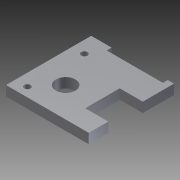
# Autodesk Inventor part: carro x lado motor pieza 2parte 2
Saved by Autodesk Inventor 2012 (Build 160160000, 160)
## iProperties
Created: 2014-12-17
Part Number: carro x lado motor pieza 2parte 2
Material: Default
Document SubType Name: Modeling
Designer: PRINCIPAL
Density: 1 g/cm^3
Author: PRINCIPAL
Autodesk Inventor part; units mm, degrees
ref_plane "YZ Plane" through (0, 0, 0) normal (1, 0, 0) x (0, 1, 0)
ref_plane "XZ Plane" through (0, 0, 0) normal (0, 1, 0) x (-1, 0, 0)
ref_plane "XY Plane" through (0, 0, 0) normal (0, 0, 1) x (1, 0, 0)
sketch "Boceto1" plane through (0, 0, 0) normal (0, 0, 1) x (1, 0, 0)
  arc A0 (-116.1173, -7.6512) -> (-117.6673, -9.2012) centre (-116.1173, -9.2012) ccw
  arc A1 (-117.6673, -9.2012) -> (-116.1173, -10.7512) centre (-116.1173, -9.2012) ccw
  arc A2 (-116.1173, -10.7512) -> (-114.5673, -9.2012) centre (-116.1173, -9.2012) ccw
  arc A3 (-114.5673, -9.2012) -> (-116.1173, -7.6512) centre (-116.1173, -9.2012) ccw
  arc A4 (-116.1173, -36.6512) -> (-117.6673, -38.2012) centre (-116.1173, -38.2012) ccw
  arc A5 (-117.6673, -38.2012) -> (-116.1173, -39.7512) centre (-116.1173, -38.2012) ccw
  arc A6 (-116.1173, -39.7512) -> (-114.5673, -38.2012) centre (-116.1173, -38.2012) ccw
  arc A7 (-114.5673, -38.2012) -> (-116.1173, -36.6512) centre (-116.1173, -38.2012) ccw
  arc A8 (-107.1173, -22.7512) -> (-112.0673, -27.7012) centre (-107.1173, -27.7012) ccw
  arc A9 (-112.0673, -27.7012) -> (-107.1173, -32.6512) centre (-107.1173, -27.7012) ccw
  arc A10 (-107.1173, -32.6512) -> (-102.1673, -27.7012) centre (-107.1173, -27.7012) ccw
  arc A11 (-102.1673, -27.7012) -> (-107.1173, -22.7512) centre (-107.1173, -27.7012) ccw
  line L0 (-122.3173, 0.4988) -> (-122.3173, -42.9012)
  line L1 (-122.3173, -42.9012) -> (-80.1673, -42.9012)
  line L2 (-80.1673, -42.9012) -> (-80.1673, -32.9643)
  line L3 (-80.1673, -32.9643) -> (-91.9173, -32.9643)
  line L4 (-91.9173, -32.9643) -> (-91.9173, -15.4172)
  line L5 (-91.9173, -15.4172) -> (-80.1673, -15.4172)
  line L6 (-80.1673, -15.4172) -> (-80.1673, 0.4988)
  line L7 (-80.1673, 0.4988) -> (-83.3173, 0.4988)
  line L8 (-83.3173, 0.4988) -> (-83.3173, -2.0012)
  line L9 (-83.3173, -2.0012) -> (-111.9173, -2.0012)
  line L10 (-111.9173, -2.0012) -> (-111.9173, 0.4988)
  line L11 (-111.9173, 0.4988) -> (-122.3173, 0.4988)
  point P0 (0, 0)
  constraints: 24 end point, 24 point on circle, 12 centre point
extrude "Extrusión1" add sketch "Boceto1" along normal blind 5
